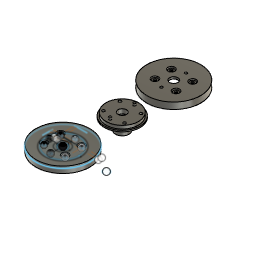
2023_05_26_V_Backup (Autodesk Fusion 360 design; units mm, degrees)
Autodesk Fusion 360 part; units mm, degrees
sketch "Sketch12" plane through (0, 0, 0) normal (0, 0, 1) x (1, 0, 0)
  circle A0 centre (0, 0) radius 22.5
  circle A1 centre (0, 0) radius 20.5
  circle A2 centre (0, 0) radius 5.25
  line L0 (0, 0) -> (0, -17) construction
  line L1 (0, 0) -> (0, -13.9) construction
  line L2 (0, -13.9) -> (0, -17) construction
  circle A3 centre (0, -15.45) radius 1.55
  circle A4 centre (0, 15.45) radius 1.55
  line L3 (0, 0) -> (-18.635, 0) construction
  line L4 (0, 0) -> (-15.225, 0) construction
  line L5 (-18.635, 0) -> (-15.225, 0) construction
  circle A5 centre (-16.93, 0) radius 1.705
  line L6 (-25, 0) -> (-25, 7.685)
  line L7 (-25, 0) -> (-25, 12.115)
  line L8 (-25, 7.685) -> (37, 7.685) construction
  line L9 (-25, 12.115) -> (37, 12.115) construction
  line L10 (0, 30) -> (-15, 30)
  line L11 (0, 30) -> (-11.3, 30)
  line L12 (-15, 30) -> (-15.225, 4.1836) construction
  line L13 (-11.3, 30) -> (-11.3, 4) construction
  circle A6 centre (-13.341, 10.4231) radius 1.705
  line L14 (-13.341, 10.4231) -> (0, 10.4231)
  line L15 (0, 10.4231) -> (-13.341, 10.4231)
  line L16 (-13.341, 10.4231) -> (-13.341, 0)
  line L17 (0, 10.4231) -> (13.341, 10.4231)
  line L18 (-13.341, 0) -> (-13.341, -10.4231)
  circle A7 centre (-13.341, -10.4231) radius 1.705
  circle A8 centre (13.341, 10.4231) radius 1.705
  line L19 (13.341, 10.4231) -> (13.341, -10.4231) construction
  circle A9 centre (13.341, -10.4231) radius 1.705
  dimension "d91" = 45
  dimension "d92" = 41
  dimension "d93" = 10.5
  dimension "d94" = 17
  dimension "d95" = 13.9
  dimension "d97" = 360
  dimension "d98" = 18.635
  dimension "d99" = 15.225
  dimension "d100" = 7.685
  dimension "d101" = 12.115
  dimension "d102" = 15
  dimension "d103" = 11.3
  dimension "d105" = 322
  constraint coincident A0.centre A1.centre
  constraint concentric A0 A1
  constraint vertical L0
  constraint parallel L0 L1
  constraint midpoint L2 A3.centre
  constraint coincident L0.end A3
  constraint perpendicular L1 L3
  constraint perpendicular L0 L4
  constraint midpoint L5 A5.centre
  constraint coincident L3.end A5
  constraint vertical L6
  constraint parallel L6 L7
  constraint perpendicular L6 L8
  constraint perpendicular L7 L9
  constraint horizontal L10
  constraint parallel L10 L11
  constraint perpendicular L8 L13
  constraint coincident A6.centre L14.start
  constraint perpendicular L13 L14
  constraint perpendicular L13 L15
  constraint vertical L16
  constraint coincident L4 L16.end
  constraint parallel L15 L17
  constraint perpendicular L4 L18
  constraint equal L14 L17
  constraint equal L16 L18
  constraint coincident L18.end A7.centre
  constraint coincident L17.end A8.centre
  constraint parallel L0 L19
  constraint coincident L19.end A9.centre
  constraint equal A6 A8
  constraint equal A6 A9
  constraint equal A6 A7
  measures "d91" diameter of A0
  measures "d92" diameter of A1
  measures "d93" diameter of A2
  measures "d94" distance of A0.centre L0.end
  measures "d95" distance of A0.centre L1.end
  measures "d98" distance of A0.centre L3.end
  measures "d99" distance of A0.centre L4.end
  measures "d100" distance of L6.start L6.end
  measures "d101" distance of L6.start L7.end
  measures "d102" distance of L10.start L10.end
  measures "d103" distance of L10.start L11.end
extrude "Extrude13" add sketch "Sketch12" against normal blind 5.7 contours A0 | A1 makes body 1
extrude "Extrude14" cut sketch "Sketch12" against normal blind 4 contours A0 bodies 1
extrude "Extrude15" add sketch "Sketch12" along normal blind -5.7 and the other way blind -2.5 contours A3 | A4 bodies 1
extrude "Extrude16" add sketch "Sketch12" against normal blind 5.7 contours A5 bodies 1
sketch "Top  Imac G4 Surface" plane through (0, 0, 0) normal (0, 0, 1) x (1, 0, 0)
  circle A0 centre (0, 0) radius 20.5
  circle A1 centre (13.341, 10.4231) radius 1.705
  circle A2 centre (-13.341, 10.4231) radius 1.705
  circle A3 centre (0, 15.45) radius 1.55
  circle A4 centre (13.341, -10.4231) radius 1.705
  circle A5 centre (0, -15.45) radius 1.55
  circle A6 centre (-13.341, -10.4231) radius 1.705
  circle A7 centre (0, 0) radius 5.25
  dimension "d117" = 41
  dimension "d118" = 10.5
  constraint equal A1 A2
  constraint equal A2 A4
  constraint equal A2 A6
  measures "d117" diameter of A0
  measures "d118" diameter of A7
sketch "Sketch14" plane through (0, 0, 0) normal (0, 0, 1) x (1, 0, 0)
  circle A0 centre (0, 0) radius 5.35
  circle A1 centre (0, 0) radius 8.5
  dimension "d119" = 10.7
  dimension "d120" = 17
  constraint coincident A0.centre A1.centre
  constraint concentric A0 A1
  measures "d119" diameter of A0
  measures "d120" diameter of A1
extrude "Extrude17" add sketch "Sketch14" against normal blind 20 bodies 1
sketch "Sketch15" plane through (0, 0, 0) normal (0, 0, 1) x (1, 0, 0)
  circle A0 centre (0, 0) radius 33.9376
  constraint coincident A0.centre origin
extrude "Extrude18" add sketch "Sketch15" along normal blind 2.5 separate body makes body 2
extrude "Extrude19" add 1 faces at (20.1568, -9.707, 0) along direction (0, 0, -1) blind 5.7 on bodies 2 bodies 2
combine "Combine3" operation cut target body 2 tool bodies 1 keep tools
extrude "Extrude20" cut 4 faces at (13.8416, -10.8224, -5.7) (13.8416, 10.0239, -5.7) (-12.8404, 10.0239, -5.7) (-12.8404, -10.8224, -5.7) along direction (0, 0, 1) blind 26 on bodies 2 bodies 2
sketch "Sketch16" plane through (0, 0, 0) normal (0, 0, 1) x (1, 0, 0)
  circle A0 centre (55, 0) radius 3.42
  circle A1 centre (55, 0) radius 1.7
  dimension "d129" = 6.84
  dimension "d130" = 3.4
  constraint concentric A0 A1
  measures "d129" diameter of A0
  measures "d130" diameter of A1
extrude "Extrude21" add sketch "Sketch16" along normal blind 5.4 separate body contours A0 | A1 makes body 3
extrude "Extrude22" cut sketch "Sketch16" along normal blind 4.3 bodies 3
draft "Draft2" angle 40 neutral plane through (0, 0, 4.3) pull (0, 0, -1) 1 faces at (58.403, -0.3405, 5.0333) on bodies 3
move_body "Move9" bodies 3 to x (1, 0, 0) y (0, 1, 0) z (0, 0, 1) at (-41.659, 10.4231, -2.9)
copy_body "CopyPasteBodies6" bodies 3 makes body 4
move_body "Move10" bodies 4 to x (1, 0, 0) y (0, 1, 0) z (0, 0, 1) at (0, -20.8463, 0)
copy_body "CopyPasteBodies7" bodies 3 4 makes body 5 makes body 6
move_body "Move11" bodies 5 6 to x (1, 0, 0) y (0, 1, 0) z (0, 0, 1) at (-26.682, 0, 0)
combine "Combine4" operation cut target body 2 tool bodies 3 4 6 5 keep tools
move_body "Move12" bodies 5 6 4 3 to x (1, 0, 0) y (0, 1, 0) z (0, 0, 1) at (0, 0, 4)
extrude "Extrude23" cut 1 faces at (-1.3756, -2.0932, -5.7) along direction (0, 0, 1) blind 25 on bodies 2 bodies 2
copy_body "CopyPasteBodies8" bodies 2 makes body 7
move_body "Move13" bodies 7 to x (1, 0, 0) y (0, 1, 0) z (0, 0, 1) at (0, 140, 0)
copy_body "CopyPasteBodies9" bodies 1 makes body 8
move_body "Move14" bodies 8 to x (1, 0, 0) y (0, 1, 0) z (0, 0, 1) at (0, 75, 0)
equation "xmax = 30 mm"
equation "xmin = 22.6 mm"
equation "ymax = 24.23 mm"
equation "ymin = 15.37 mm"
equation "middlemin = 27.8 mm"
equation "middlemax = 34 mm"
equation "d94 = middlemax / 2"
equation "d95 = middlemin / 2"
equation "d98 = 37.27 mm / 2"
equation "d99 = ( 30.45 / 2 ) * 1 mm"
equation "d100 = ymin / 2"
equation "d101 = ymax / 2"
equation "d102 = xmax / 2"
equation "d103 = ( xmin / 2 mm ) * 1 mm"
equation "ScrewDim = 3.5 mm"
equation "d109 = -5.70 mm + 1.7 mm"
equation "d133 = 5.40 mm - 1.1 mm"
named bodies: "Top Imac G4 Part", "Toop Imac G4 wrapper", "Toop Imac G4 wrapper (1)", "Top Imac G4 Part (1)"
